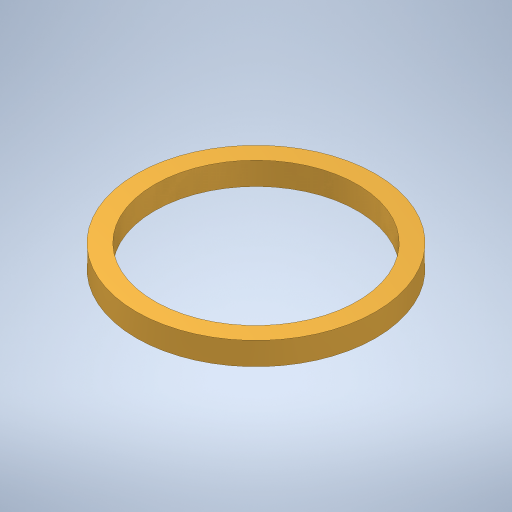
# Autodesk Inventor part: press
Saved by Autodesk Inventor 2024 (Build 280153000, 153)
## iProperties
Created: 2023-11-04
Part Number: press
Material: Brass, Soft Yellow
Document SubType Name: Modeling
Designer: schanen
Density: 8.47 g/cm^3
Appearance: Brass - Satin
Author: schanen
Autodesk Inventor part; units mm, degrees
ref_plane "YZ Plane" through (0, 0, 0) normal (1, 0, 0) x (0, 1, 0)
ref_plane "XZ Plane" through (0, 0, 0) normal (0, 1, 0) x (-1, 0, 0)
ref_plane "XY Plane" through (0, 0, 0) normal (0, 0, 1) x (1, 0, 0)
sketch "Sketch1" plane through (0, 0, 0) normal (0, 0, 1) x (1, 0, 0)
  line L0 (-22.225, 0) -> (-26.225, 0)
  line L1 (-26.225, 0) -> (-26.225, 5)
  line L2 (-26.225, 5) -> (-22.225, 5)
  line L3 (-22.225, 5) -> (-22.225, 0)
  line L4 (0, -1) -> (0, 6) projected
  point P0 (0, 0)
  dimension "d0" = 22.225
  dimension "d1" = 5
  dimension "d2" = 4
  constraints: 8 end point, 2 parallel, 1 horizontal, 1 horizontal alignment, 1 perpendicular
  measures "d0" distance from line of point (0, 0) L3
  measures "d1" distance of L2.end L0.start
  measures "d2" distance of L1.end L2.end
revolve "Revolution1" add sketch "Sketch1" angle 360 about axis through (0, -10, 0) along (0, 1, 0)
equation "\"d0\" = 0.5 * cylinder_od"
equation "\"d2\" = oring_dia"
equation "\"oring_dia\" = 4"
equation "\"cylinder_od\" = 44.45"
body "Solid1"
